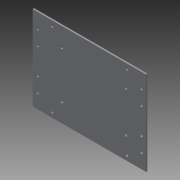
# Autodesk Inventor part: バッテリー固定
Saved by Autodesk Inventor 2014 (Build 180170000, 170)
## iProperties
Created: 2013-09-12
Part Number: バッテリー固定
Material: 一般
Document SubType Name: Modeling
Designer: koki
Density: 1 g/cm^3
Appearance: 既定
Author: koki
Autodesk Inventor part; units mm, degrees
ref_plane "YZ Plane" through (0, 0, 0) normal (1, 0, 0) x (0, 1, 0)
ref_plane "XZ Plane" through (0, 0, 0) normal (0, 1, 0) x (-1, 0, 0)
ref_plane "XY Plane" through (0, 0, 0) normal (0, 0, 1) x (1, 0, 0)
sketch "スケッチ1" plane through (0, 0, 0) normal (0, 1, 0) x (-1, 0, 0)
  line L0 (-20.4773, 9.5578) -> (96.5227, 9.5578)
  line L1 (96.5227, 9.5578) -> (96.5227, -77.4422)
  line L2 (96.5227, -77.4422) -> (-20.4773, -77.4422)
  line L3 (-20.4773, -77.4422) -> (-20.4773, 9.5578)
  point P0 (0, 0)
  dimension "d0" = 117
  dimension "d1" = 87
  constraints: 8 end point, 2 parallel, 1 horizontal, 1 perpendicular
  measures "d0" distance of L1.end L2.end
  measures "d1" distance of L0.end L1.end
extrude "押し出し1" add sketch "スケッチ1" along normal blind 1.5
sketch "スケッチ2" plane through (0, 1.5, 0) normal (0, 1, 0) x (1, 0, 0)
  line L0 (-96.5227, -9.5578) -> (20.4773, -9.5578) projected
  line L1 (20.4773, -9.5578) -> (20.4773, 77.4422) projected
  line L2 (20.4773, 77.4422) -> (-96.5227, 77.4422) projected
  line L3 (-96.5227, 77.4422) -> (-96.5227, -9.5578) projected
  point P0 (0, 0)
  point P1 (-76.5227, 72.4422)
  point P2 (0.4773, 72.4422)
  point P3 (-76.5227, -4.5578)
  point P4 (0.4773, -4.5578)
  dimension "d4" = 5
  dimension "d5" = 5
  dimension "d6" = 5
  dimension "d7" = 5
  dimension "d8" = 20
  dimension "d9" = 20
  dimension "d10" = 20
  dimension "d11" = 20
  measures "d4" distance from line of L2 point (-76.523, 72.442)
  measures "d5" distance from line of L2 point (0.477, 72.442)
  measures "d6" distance from line of L0 point (-76.523, -4.558)
  measures "d7" distance from line of L0 point (0.477, -4.558)
  measures "d8" distance from line of L3 point (-76.523, 72.442)
  measures "d9" distance from line of L1 point (0.477, 72.442)
  measures "d10" distance from line of L3 point (-76.523, -4.558)
  measures "d11" distance from line of L1 point (0.477, -4.558)
hole "穴1" at (-76.5227, 1.5, -72.4422) at (0.4773, 1.5, -72.4422) at (-76.5227, 1.5, 4.5578) at (0.4773, 1.5, 4.5578) direction (0, -1, 0) diameter 3 end through all
sketch "スケッチ3" plane through (0, 1.5, 0) normal (0, 1, 0) x (1, 0, 0)
  line L0 (-96.5227, -9.5578) -> (20.4773, -9.5578) projected
  line L1 (20.4773, -9.5578) -> (20.4773, 77.4422) projected
  line L2 (20.4773, 77.4422) -> (-96.5227, 77.4422) projected
  line L3 (-96.5227, 77.4422) -> (-96.5227, -9.5578) projected
  point P0 (0, 0)
  point P1 (-91.5227, 47.4422)
  point P2 (-91.5227, 47.4422)
  point P3 (-91.5227, 62.4422)
  point P4 (-91.5227, 20.4422)
  point P5 (-91.5227, 5.4422)
  point P6 (15.4773, 62.4422)
  point P7 (15.4773, 47.4422)
  point P8 (15.4773, 20.4422)
  point P9 (15.4773, 5.4422)
  dimension "d19" = 5
  dimension "d20" = 5
  dimension "d21" = 5
  dimension "d22" = 5
  dimension "d23" = 30
  dimension "d24" = 15
  dimension "d25" = 15
  dimension "d26" = 30
  dimension "d27" = 15
  dimension "d28" = 30
  dimension "d29" = 15
  dimension "d30" = 30
  dimension "d31" = 5
  dimension "d32" = 5
  dimension "d33" = 5
  dimension "d34" = 5
  constraints: 1 coincident
  measures "d19" distance from line of L3 point (-91.523, 47.442)
  measures "d20" distance from line of L3 point (-91.523, 62.442)
  measures "d21" distance from line of L3 point (-91.523, 20.442)
  measures "d22" distance from line of L3 point (-91.523, 5.442)
  measures "d23" distance from line of L2 point (-91.523, 47.442)
  measures "d24" distance from line of L2 point (-91.523, 62.442)
  measures "d25" distance from line of L0 point (-91.523, 5.442)
  measures "d26" distance from line of L0 point (-91.523, 20.442)
  measures "d27" distance from line of L2 point (15.477, 62.442)
  measures "d28" distance from line of L2 point (15.477, 47.442)
  measures "d29" distance from line of L0 point (15.477, 5.442)
  measures "d30" distance from line of L0 point (15.477, 20.442)
  measures "d31" distance from line of L1 point (15.477, 62.442)
  measures "d32" distance from line of L1 point (15.477, 47.442)
  measures "d33" distance from line of L1 point (15.477, 20.442)
  measures "d34" distance from line of L1 point (15.477, 5.442)
hole "穴2" at (-91.5227, 1.5, -47.4422) at (-91.5227, 1.5, -62.4422) at (-91.5227, 1.5, -20.4422) at (-91.5227, 1.5, -5.4422) at (15.4773, 1.5, -62.4422) at (15.4773, 1.5, -47.4422) at (15.4773, 1.5, -20.4422) at (15.4773, 1.5, -5.4422) direction (0, -1, 0) diameter 3 end through all
sketch "スケッチ4" plane through (0, 1.5, 0) normal (0, 1, 0) x (1, 0, 0)
  line L0 (20.4773, -9.5578) -> (20.4773, 77.4422) projected
  line L1 (20.4773, 77.4422) -> (-96.5227, 77.4422) projected
  line L2 (5.1573, 61.2472) -> (-81.2027, 61.2472)
  line L3 (-81.2027, 61.2472) -> (-81.2027, 6.6372)
  line L4 (-81.2027, 61.2472) -> (5.1573, 61.2472)
  line L5 (5.1573, 6.6372) -> (-81.2027, 6.6372)
  line L6 (-81.2027, 6.6372) -> (-81.2027, 61.2472)
  line L7 (-81.2027, 6.6372) -> (5.1573, 6.6372)
  line L8 (5.1573, 6.6372) -> (5.1573, 61.2472)
  point P0 (-96.5227, -9.5578)
  point P1 (0, 0)
  point P2 (0, 0)
  point P3 (0, 0)
  point P4 (-0.5577, 54.8972)
  point P5 (-0.5577, 12.9872)
  point P6 (-66.5977, 9.8122)
  point P7 (-66.5977, 58.0722)
  dimension "d42" = 86.36
  dimension "d43" = 54.61
  dimension "d44" = 14.605
  dimension "d45" = 3.175
  dimension "d46" = 3.175
  dimension "d47" = 14.605
  dimension "d48" = 6.35
  dimension "d50" = 6.35
  dimension "d52" = 0
  dimension "d53" = 0
  dimension "d54" = 87
  dimension "d55" = 16.195
  dimension "d56" = 117
  dimension "d58" = 15.32
  dimension "d59" = 5.715
  dimension "d60" = 5.715
  dimension "d61" = 66.04
  dimension "d62" = 66.04
  constraints: 14 end point, 1 horizontal, 1 parallel
  measures "d42" distance of L5.start L5.end
  measures "d43" distance of L4.end L5.start
  measures "d44" distance from line of L6 point (-66.598, 58.072)
  measures "d45" distance from line of L4 point (-66.598, 58.072)
  measures "d46" distance from line of L5 point (-66.598, 9.812)
  measures "d47" distance from line of L6 point (-66.598, 9.812)
  measures "d48" distance from line of L5 point (-0.558, 12.987)
  measures "d50" distance from line of L4 point (-0.558, 54.897)
  measures "d52" distance between parallel lines of L2 L4
  measures "d53" distance between parallel lines of L3 L6
  measures "d54" distance of L0.start L0.end
  measures "d55" distance between parallel lines of L1 L2
  measures "d56" distance of point (-96.523, -9.558) L0.start
  measures "d58" distance between parallel lines of L0 L8
  measures "d59" distance from line of L8 point (-0.558, 54.897)
  measures "d60" distance from line of L8 point (-0.558, 12.987)
  measures "d61" horizontal distance of point (-66.598, 9.812) point (-0.558, 12.987)
  measures "d62" horizontal distance of point (-66.598, 58.072) point (-0.558, 54.897)
hole "穴3" at (-66.5977, 1.5, -58.0722) at (-66.5977, 1.5, -9.8122) at (-0.5577, 1.5, -12.9872) at (-0.5577, 1.5, -54.8972) direction (0, -1, 0) diameter 3 end through all
equation "\"d5\" = d4"
equation "\"d6\" = d4"
equation "\"d7\" = d6"
equation "\"d9\" = d8"
equation "\"d10\" = d8"
equation "\"d11\" = d9"
equation "\"d20\" = d19"
equation "\"d21\" = d20"
equation "\"d22\" = d20"
equation "\"d32\" = d31"
equation "\"d33\" = d32"
equation "\"d34\" = d33"
equation "\"d55\" = 0.5 * d54 - 0.5 * d43"
equation "\"d58\" = 0.5 * d56 - 0.5 * d42"
